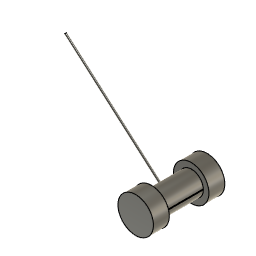
Auto_CatStick_shell v1 (Autodesk Fusion 360 design; units mm, degrees)
Autodesk Fusion 360 part; units mm, degrees
cylinder "CylinderPrimitive1" add diameter 60 height 100 placed x (1, 0, 0) y (0, 0, -1) z (0, 1, 0) at (5, 0, 15) makes body 1
hole "Hole1" at (5.2686, 100, 14.685) direction (0, -1, 0) diameter 50 depth 100 tip angle 180 bodies 1
box "BoxPrimitive2" add length 100 width 39 height 2 placed x (0, 1, 0) y (-1, 0, 0) z (0, 0, 1) at (25, -0.8478, 0) separate body makes body 2
move_body "Move1" bodies 2 to x (1, 0, 0) y (0, 1, 0) z (0, 0, 1) at (0, 0, 15)
extrude "Extrude1" add 1 faces at (25, 32.4855, 15.6667) along direction (1, 0, 0) blind 10 on bodies 2 bodies 2 1
extrude "Extrude2" cut 1 faces at (-14, 32.4855, 15.6667) along direction (-1, 0, 0) blind 10 on bodies 2 bodies 2
extrude "Extrude3" add 1 faces at (-14, 32.4855, 15.6667) along direction (-1, 0, 0) blind 10 on bodies 2 bodies 2
cylinder "CylinderPrimitive3" add diameter 89.443 height 20 placed x (1, 0, 0) y (0, 0, -1) z (0, 1, 0) at (345, 0, 470) separate body makes body 3
move_body "Move3" bodies 3 to x (1, 0, 0) y (0, 1, 0) z (0, 0, 1) at (-340.6581, -25, -455.4141)
move_body "Move4" bodies 3 to x (1, 0, 0) y (0, 1, 0) z (0, 0, 1) at (0, 5, 0)
copy_body "CopyPasteBodies1" bodies 3 makes body 4
move_body "Move5" bodies 4 to x (1, 0, 0) y (0, 1, 0) z (0, 0, 1) at (0, 120, 0)
extrude "Extrude4" add 1 faces at (-7.975, 120, 6.1883) along direction (0, 1, 0) blind 20 on bodies 4 bodies 4
extrude "Extrude5" add 1 faces at (-7.975, -20, 6.1883) along direction (0, -1, 0) blind 20 on bodies 3 bodies 3
cylinder "CylinderPrimitive4" add diameter 5 height 325 placed x (1, 0, 0) y (0, 0, -1) z (0, 1, 0) at (-90, 0, 25) separate body makes body 5
move_body "Move6" bodies 5 to x (-0.265464, 0.878005, -0.39829) y (-0.80017, 0.029809, 0.599032) z (0.537826, 0.477722, 0.69464) at (-100.0836, 389.2453, 55.6774)
move_body "Move7" bodies 5 to x (1, 0, 0) y (0, 1, 0) z (0, 0, 1) at (67.8527, -277.6996, -62.4814)
move_body "Move8" bodies 5 to x (0.996422, -0.025976, -0.080429) y (0.033086, 0.995537, 0.088381) z (0.077774, -0.090726, 0.992834) at (-23.9891, 6.2721, -26.4897)
form "Form1" [no effect]
